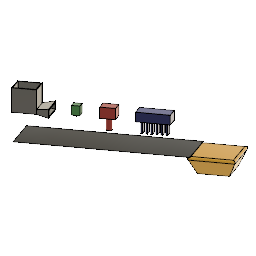
ChopperSubsystemRoughOutlineV1 (Autodesk Fusion 360 design; units mm, degrees)
Autodesk Fusion 360 part; units mm, degrees
sketch "ConveryorBelt" plane through (0, 0, 0) normal (0, 0, 1) x (1, 0, 0)
  line L0 (-1500, 1000) -> (5550, 1000)
  line L1 (5550, 1000) -> (5550, -1000)
  line L2 (5550, -1000) -> (-1500, -1000)
  line L3 (-1500, -1000) -> (-1500, 1000)
  dimension "d1" = 7050
  dimension "d2" = 2000
  constraint horizontal L0
  constraint vertical L1
  constraint horizontal L2
  constraint vertical L3
  measures "d1" distance of L0.start L0.end
  measures "d2" distance of L0.end L1.end
sketch "VegetableStorage/Dropping" plane through (0, 0, 0) normal (0, 0, 1) x (1, 0, 0)
  line L0 (-1700, 416.3983) -> (-702.4107, 416.3983)
  line L1 (-702.4107, 416.3983) -> (-702.4107, -450)
  line L2 (-702.4107, -450) -> (-1700, -450)
  line L3 (-1700, -450) -> (-1700, 416.3983)
  constraint horizontal L0
  constraint vertical L1
  constraint horizontal L2
  constraint vertical L3
extrude "Extrude1" add sketch "ConveryorBelt" along normal blind 3 makes body 1
extrude "Extrude2" add sketch "VegetableStorage/Dropping" along normal blind 1000 from surface at 1000 separate body makes body 2
shell "Shell1" thickness 40 removed faces 1 at (-1367.4702, 127.5989, 2000) on bodies 2
sketch "VegetableStorageProtrusion" plane through (-702.4107, 0, 0) normal (1, 0, 0) x (0, 1, 0)
  line L0 (-450, 1000) -> (416.3983, 1000)
  line L1 (416.3983, 1000) -> (416.3983, 2000)
  line L2 (416.3983, 2000) -> (-450, 2000)
  line L3 (-450, 2000) -> (-450, 1000)
  line L4 (-450, 1200) -> (416.3983, 1200)
  line L5 (416.3983, 1200) -> (416.3983, 1000)
  line L6 (416.3983, 1000) -> (-450, 1000)
  line L7 (-450, 1000) -> (-450, 1200)
  constraint horizontal L4
  constraint vertical L5
  constraint horizontal L6
  constraint vertical L7
  constraint collinear L1 L5
  constraint collinear L3 L7
  constraint collinear L0 L6
extrude "Extrude3" add sketch "VegetableStorageProtrusion" along normal blind 500 draft 10 contours L0 L1 L3 L4 L5 L6 L7 bodies 2
shell "Shell2" thickness 60 removed faces 1 at (-202.4107, 156.9867, 1037.2788) on bodies 2
sketch "ComputerVisionCamera" plane through (0, 0, 3) normal (0, 0, 1) x (-1, 0, 0)
  line L0 (1500, 1000) -> (-5550, 1000)
  line L1 (-5550, 1000) -> (-5550, -1000)
  line L2 (-5550, -1000) -> (1500, -1000)
  line L3 (1500, -1000) -> (1500, 1000)
  line L4 (-600, -172.6758) -> (-947.5188, -172.6758)
  line L5 (-947.5188, -172.6758) -> (-947.5188, 174.843)
  line L6 (-947.5188, 174.843) -> (-600, 174.843)
  line L7 (-600, 174.843) -> (-600, -172.6758)
  constraint horizontal L4
  constraint vertical L5
  constraint horizontal L6
  constraint vertical L7
  constraint equal L5 L6
extrude "Extrude5" add sketch "ComputerVisionCamera" along normal blind 400 from surface at 1000 separate body contours L4 L5 L6 L7 makes body 3
sketch "CameraExtension" plane through (0, 0, 1003) normal (0, 0, -1) x (1, 0, 0)
  line L0 (947.5188, 174.843) -> (600, 174.843)
  line L1 (600, 174.843) -> (600, -172.6758)
  line L2 (600, -172.6758) -> (947.5188, -172.6758)
  line L3 (947.5188, -172.6758) -> (947.5188, 174.843)
  circle A0 centre (773.7594, 1.0836) radius 77.5643
  line L4 (773.7594, 174.843) -> (773.7594, -172.6758)
  point P0 (773.7594, 1.0836)
  constraint midpoint L0 L4.start
  constraint midpoint L2 L4.end
  constraint midpoint L4 P0
  constraint coincident P0 A0.centre
extrude "Extrude6" add sketch "CameraExtension" along normal blind 60 contours A0 L4 | A0 L4 bodies 3
sketch "PrepMachine" plane through (0, 0, 3) normal (0, 0, 1) x (-1, 0, 0)
  line L0 (1500, 1000) -> (-5550, 1000)
  line L1 (-5550, 1000) -> (-5550, -1000)
  line L2 (-5550, -1000) -> (1500, -1000)
  line L3 (1500, -1000) -> (1500, 1000)
  line L4 (202.4107, -443.6362) -> (202.4107, 477.2379)
  line L5 (-1749.5188, -250) -> (-2387.8803, -250)
  line L6 (-2387.8803, -250) -> (-2387.8803, 250)
  line L7 (-2387.8803, 250) -> (-1749.5188, 250)
  line L8 (-1749.5188, 250) -> (-1749.5188, -250)
  line L9 (-947.5188, -172.6758) -> (-947.5188, 174.843)
  point P0 (-600, -172.6758)
  constraint horizontal L5
  constraint vertical L6
  constraint horizontal L7
  constraint vertical L8
extrude "Extrude8" add sketch "PrepMachine" along normal blind 460 from surface at 1000 separate body contours L5 L6 L7 L8 makes body 4
sketch "PrepMachine-Decore" plane through (0, 0, 1003) normal (0, 0, -1) x (1, 0, 0)
  line L0 (2387.8803, 250) -> (1749.5188, 250)
  line L1 (1749.5188, 250) -> (1749.5188, -250)
  line L2 (1749.5188, -250) -> (2387.8803, -250)
  line L3 (2387.8803, -250) -> (2387.8803, 250)
  circle A0 centre (2068.6995, -1.0765) radius 122.2133
  circle A1 centre (2068.6995, -1.0765) radius 80.1333
  constraint concentric A0 A1
extrude "Extrude9" add sketch "PrepMachine-Decore" along normal blind 520 contours A0 bodies 4
fillet "Fillet1" radius 15 1 edges at (701.4441, 26.9648, 943) on bodies 3
sketch "Chopper" plane through (0, 0, 3) normal (0, 0, 1) x (-1, 0, 0)
  line L0 (-3189.8803, -300) -> (-4580.7729, -300)
  line L1 (-4580.7729, -300) -> (-4580.7729, 300)
  line L2 (-4580.7729, 300) -> (-3189.8803, 300)
  line L3 (-3189.8803, 300) -> (-3189.8803, -300)
  line L4 (-2387.8803, -250) -> (-2387.8803, 250)
  constraint horizontal L0
  constraint vertical L1
  constraint horizontal L2
  constraint vertical L3
extrude "Extrude10" add sketch "Chopper" along normal blind 400 from surface at 1000 separate body makes body 5
sketch "ChopperBlades" plane through (0, 0, 1003) normal (0, 0, -1) x (1, 0, 0)
  line L0 (4580.7729, 300) -> (3189.8803, 300)
  line L1 (3189.8803, 300) -> (3189.8803, -300)
  line L2 (3189.8803, -300) -> (4580.7729, -300)
  line L3 (4580.7729, -300) -> (4580.7729, 300)
  line L4 (4432.8571, 150) -> (4362.8571, 150)
  line L5 (4362.8571, 150) -> (4362.8571, -150)
  line L6 (4362.8571, -150) -> (4432.8571, -150)
  line L7 (4432.8571, -150) -> (4432.8571, 150)
  line L8 (4232.8571, 150) -> (4162.8571, 150)
  line L9 (4162.8571, 150) -> (4162.8571, -150)
  line L10 (4162.8571, -150) -> (4232.8571, -150)
  line L11 (4232.8571, -150) -> (4232.8571, 150)
  line L12 (4032.8571, 150) -> (3962.8571, 150)
  line L13 (3962.8571, 150) -> (3962.8571, -150)
  line L14 (3962.8571, -150) -> (4032.8571, -150)
  line L15 (4032.8571, -150) -> (4032.8571, 150)
  line L16 (3832.8571, 150) -> (3762.8571, 150)
  line L17 (3762.8571, 150) -> (3762.8571, -150)
  line L18 (3762.8571, -150) -> (3832.8571, -150)
  line L19 (3832.8571, -150) -> (3832.8571, 150)
  line L20 (3632.8571, 150) -> (3562.8571, 150)
  line L21 (3562.8571, 150) -> (3562.8571, -150)
  line L22 (3562.8571, -150) -> (3632.8571, -150)
  line L23 (3632.8571, -150) -> (3632.8571, 150)
  line L24 (3432.8571, 150) -> (3362.8571, 150)
  line L25 (3362.8571, 150) -> (3362.8571, -150)
  line L26 (3362.8571, -150) -> (3432.8571, -150)
  line L27 (3432.8571, -150) -> (3432.8571, 150)
  constraint horizontal L4
  constraint vertical L5
  constraint horizontal L6
  constraint vertical L7
  constraint horizontal L8
  constraint vertical L9
  constraint horizontal L10
  constraint vertical L11
  constraint horizontal L12
  constraint vertical L13
  constraint horizontal L14
  constraint vertical L15
  constraint horizontal L16
  constraint vertical L17
  constraint horizontal L18
  constraint vertical L19
  constraint horizontal L20
  constraint vertical L21
  constraint horizontal L22
  constraint vertical L23
  constraint horizontal L24
  constraint vertical L25
  constraint horizontal L26
  constraint vertical L27
  constraint equal L20 L24
  constraint equal L16 L24
  constraint equal L12 L24
  constraint equal L8 L24
  constraint equal L4 L24
extrude "Extrude11" add sketch "ChopperBlades" along normal blind 500 contours L4 L5 L6 L7 | L8 L9 L10 L11 | L12 L13 L14 L15 | L16 L17 L18 L19 | L20 L21 L22 L23 | L24 L25 L26 L27 bodies 5
sketch "ChoppedVeggieCollector" plane through (0, 0, 0) normal (0, 0, 1) x (1, 0, 0)
  line L0 (5400.7729, 989.9184) -> (7380.6099, 989.9184)
  line L1 (7380.6099, 989.9184) -> (7380.6099, -989.9186)
  line L2 (7380.6099, -989.9186) -> (5400.7729, -989.9186)
  line L3 (5400.7729, -989.9186) -> (5400.7729, 989.9184)
  line L4 (4580.7729, 300) -> (4580.7729, -300)
  line L5 (5400.7729, 989.9184) -> (7380.6099, -989.9186)
  line L6 (7380.6099, 989.9184) -> (5400.7729, -989.9186)
  line L7 (1.75, 0) -> (22.5, 0)
  point P0 (6390.6914, -0.0001)
  constraint horizontal L0
  constraint vertical L1
  constraint horizontal L2
  constraint vertical L3
  constraint perpendicular L5 L6
  constraint midpoint L5 P0
extrude "Extrude12" add sketch "ChoppedVeggieCollector" along normal blind 0 draft 20 and the other way blind 750 draft -25 separate body makes body 6
fillet "Fillet2" radius 90 1 faces at (6060.7186, 329.9727, 0) on bodies 6
named bodies: "ConveyorBElt", "VegetableStorer/Dropper", "ComputerVisionCamera", "Prep&Decore", "Chopper", "ChoppedVeggieCollector"
